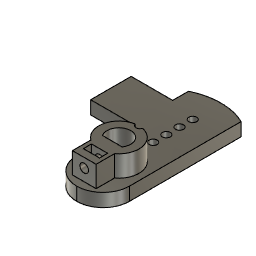
partA_5-1_geared v8 (Autodesk Fusion 360 design; units mm, degrees)
Autodesk Fusion 360 part; units mm, degrees
note: some values were not read from the file. Chosen so that the rebuilt part matches the saved one: which face or edge a step refers to. Set by a fixed rule: which sketch regions a step uses.
sketch "Sketch1" plane through (0, 0, 0) normal (0, 0, 1) x (1, 0, 0)
  circle A0 centre (19.9632, 20.0536) radius 32
  circle A1 centre (19.9632, 20.0536) radius 2.5692
  line L0 (16.8979, 9.6411) -> (23.0286, 9.6411)
  line L1 (23.0286, 9.6411) -> (23.0286, 12.7065)
  line L2 (23.0286, 12.7065) -> (16.8979, 12.7065)
  line L3 (16.8979, 12.7065) -> (16.8979, 9.6411)
  line L4 (18.9305, 17.7012) -> (20.996, 17.7012)
  circle A2 centre (20.0539, 47.9478) radius 1.5
  line L5 (19.9632, 20.0536) -> (20.0539, 47.9478) construction
  circle A3 centre (20.0539, 42.9478) radius 1.5
  circle A4 centre (20.0539, 37.9478) radius 1.5
  circle A5 centre (20.0539, 32.9478) radius 1.5
  circle A6 centre (20.0539, 27.9478) radius 1.5
  circle A7 centre (19.9632, 20.0536) radius 4.5
  line L6 (19.9779, 24.5536) -> (19.9551, 17.5536) construction
  line L7 (19.9551, 17.5536) -> (16.2135, 17.5658)
  line L8 (19.9551, 17.5536) -> (23.6968, 17.5415)
  dimension "d1" = 64
  dimension "d2" = 3
  dimension "d18" = 3
  dimension "d19" = 3
  dimension "d20" = 3
  dimension "d21" = 3
  dimension "d26" = 9
  dimension "d27" = 7
  constraint concentric A0 A1
  constraint horizontal L0
  constraint vertical L1
  constraint horizontal L2
  constraint vertical L3
  constraint coincident A1 L4.start
  constraint coincident A1 L4.end
  constraint horizontal L4
  constraint coincident A0.centre A1.centre
  constraint coincident A2.centre L5.end
  constraint concentric A0 A7
  constraint coincident A7 L6.start
  constraint coincident L5 L6.start
  constraint parallel L5 L6
  constraint coincident A7 L7.end
  constraint perpendicular L6 L7
  constraint coincident A7 L8.end
  constraint perpendicular L6 L8
  measures "d1" diameter of A0
  measures "d2" diameter of A2
  measures "d18" diameter of A3
  measures "d19" diameter of A4
  measures "d20" diameter of A5
  measures "d21" diameter of A6
  measures "d26" diameter of A7
  measures "d27" distance of L6.start L6.end
extrude "Extrude1" add sketch "Sketch1" along normal blind 5 contours A0 | A1 A7 L7 L8 | A1 L4 L7 L8 | A1 L7 L8 | A1 A7 L7 L8 | A3 | A4 | A5 | A6
sketch "Sketch2" plane through (0, 0, 5) normal (0, 0, 1) x (-1, 0, 0)
  line L0 (-20.996, -17.7012) -> (-18.9305, -17.7012)
  arc A0 (-20.996, -17.7012) -> (-18.9305, -17.7012) centre (-19.9632, -20.0536) ccw
  circle A1 centre (-20.0539, -47.9478) radius 1.5
  line L1 (-16.8979, -9.6411) -> (-16.8979, -12.7065)
  line L2 (-16.8979, -12.7065) -> (-23.0286, -12.7065)
  line L3 (-23.0286, -12.7065) -> (-23.0286, -9.6411)
  line L4 (-23.0286, -9.6411) -> (-16.8979, -9.6411)
  circle A2 centre (-19.9632, -20.0536) radius 32
  circle A3 centre (-19.9632, -20.0536) radius 7.6208
  line L5 (-15.4848, -13.8875) -> (-24.4668, -13.8875)
  line L6 (-24.4668, -13.8875) -> (-24.4668, -6.9024)
  line L7 (-24.4668, -6.9024) -> (-15.4848, -6.9024)
  line L8 (-15.4848, -6.9024) -> (-15.4848, -13.8875)
  line L9 (-16.8979, -12.7065) -> (-23.0286, -12.7065)
  line L10 (-23.0286, -12.7065) -> (-23.0286, -13.8875)
  line L11 (-23.0286, -13.8875) -> (-16.8979, -13.8875)
  line L12 (-16.8979, -13.8875) -> (-16.8979, -12.7065)
  constraint concentric A0 A3
  constraint horizontal L5
  constraint vertical L6
  constraint horizontal L7
  constraint vertical L8
  constraint coincident A3 L5.start
  constraint horizontal L9
  constraint vertical L10
  constraint horizontal L11
  constraint vertical L12
  constraint coincident L5 L10.end
  constraint coincident L3 L10.end
  constraint coincident L1.end L2.start
extrude "Extrude2" add sketch "Sketch2" along normal blind 10 contours L1 L3 L4 A3 L5 L6 L7 L8 L10 L12 | L1 L2 L3 L4 A3 L9 | L2 A3 L9 L12 | L2 A3 L5 L9 L10 L11 L12 | A3 L5 L12 | L2 A3 L9 L10 | A3 L5 L11 | A3 L5 L10
sketch "Sketch3" plane through (0, 6.9024, 0) normal (0, -1, 0) x (1, 0, 0)
  line L0 (15.4848, 5) -> (24.4668, 5)
  line L1 (24.4668, 5) -> (24.4668, 15)
  line L2 (24.4668, 15) -> (15.4848, 15)
  line L3 (15.4848, 15) -> (15.4848, 5)
  circle A0 centre (19.9584, 9.4906) radius 1.65
  dimension "d7" = 3.3
  measures "d7" diameter of A0
extrude "Extrude3" cut sketch "Sketch3" against normal up to surface (10.7988 mm away) contours A0
sketch "Sketch4" plane through (0, 0, 0) normal (0, 0, -1) x (1, 0, 0)
  line L0 (18.9305, -17.7012) -> (20.996, -17.7012)
  arc A0 (18.9305, -17.7012) -> (20.996, -17.7012) centre (19.9632, -20.0536) ccw
  circle A1 centre (20.0539, -47.9478) radius 1.5
  line L1 (16.8979, -12.7065) -> (16.8979, -9.6411)
  line L2 (16.8979, -9.6411) -> (23.0286, -9.6411)
  line L3 (23.0286, -9.6411) -> (23.0286, -12.7065)
  line L4 (23.0286, -12.7065) -> (16.8979, -12.7065)
  circle A2 centre (19.9632, -20.0536) radius 32
  line L5 (19.9632, -20.0536) -> (19.9632, -4.0536) construction
  line L6 (19.9632, -4.0536) -> (29.9632, -4.0536)
  line L7 (29.9632, -4.0536) -> (29.9333, -50.4608)
  line L8 (9.9632, -4.0536) -> (9.9932, -50.4608)
  line L9 (19.9632, -4.0536) -> (9.9632, -4.0536)
  dimension "d10" = 16
  dimension "d11" = 10
  constraint coincident A0.centre A2.centre
  constraint perpendicular L2 L5
  constraint perpendicular L5 L6
  constraint coincident A2 L7.end
  constraint symmetric L6.start L5 L9.start
  constraint symmetric L5 L6.end L8.start
  constraint symmetric L5 L7.end L8.end
  measures "d10" distance of A0.centre L5.end
  measures "d11" distance of L5.end L6.end
extrude "Extrude4" cut sketch "Sketch4" against normal blind 17 contours A2 L6 L7 L8 L9 picked at (14.6424, 1.0929)
fillet "Fillet1" radius 10 2 edges at (9.9632, 4.0536, 2.5) (29.9632, 4.0536, 2.5)
fillet "Fillet2" radius 4 2 edges at (29.9333, 50.4608, 2.5) (9.9932, 50.4608, 2.5)
extrude "Extrude5" cut sketch "Sketch1" along normal up to surface (5 mm away) contours A3 | A4 | A5 | A6
extrude "Extrude6" cut sketch "Sketch1" along normal blind 16 contours A6
extrude "Extrude7" cut sketch "Sketch1" along normal up to surface (15 mm away) contours A1 L4 | A1 A7 L7 L8 | A1 L4 L7 L8 picked at (16.6304, 18.132)
sketch "Sketch5" plane through (0, 0, 15) normal (0, 0, 1) x (-1, 0, 0)
  line L0 (-23.6968, -17.5415) -> (-16.2135, -17.5658)
  arc A0 (-23.6968, -17.5415) -> (-16.2135, -17.5658) centre (-19.9632, -20.0536) ccw
  arc A1 (-18.6069, -27.5528) -> (-21.4915, -27.5196) centre (-20.0539, -27.9478) ccw
  arc A2 (-18.6069, -27.5528) -> (-15.4848, -13.8875) centre (-19.9632, -20.0536) ccw
  line L1 (-15.4848, -13.8875) -> (-15.4848, -6.9024)
  line L2 (-15.4848, -6.9024) -> (-24.4668, -6.9024)
  line L3 (-24.4668, -6.9024) -> (-24.4668, -13.8875)
  line L4 (-24.4668, -13.8875) -> (-24.4417, -13.8875)
  arc A3 (-24.4417, -13.8875) -> (-21.4915, -27.5196) centre (-19.9632, -20.0536) ccw
  arc A4 (-17.9394, -12.7065) -> (-21.9871, -12.7065) centre (-19.9632, -20.0536) ccw
  line L5 (-17.9394, -12.7065) -> (-21.9871, -12.7065)
  line L6 (-17.9394, -12.7065) -> (-21.9871, -12.7065)
  arc A5 (-17.9394, -12.7065) -> (-21.9871, -12.7065) centre (-19.9632, -20.0536) ccw
  constraint coincident A4.start L5.start
  constraint coincident A4.end L5.end
extrude "Extrude8" add sketch "Sketch5" against normal blind 15 contours A4 L5 L6 A5
sketch "Sketch6" plane through (0, 0, 0) normal (0, 0, -1) x (1, 0, 0)
  line L0 (16.2135, -17.5658) -> (23.6968, -17.5415)
  arc A0 (16.2135, -17.5658) -> (23.6968, -17.5415) centre (19.9632, -20.0536) ccw
  circle A1 centre (20.0539, -37.9478) radius 1.5
  circle A2 centre (20.0539, -32.9478) radius 1.5
  circle A3 centre (20.0539, -42.9478) radius 1.5
  circle A4 centre (20.0539, -27.9478) radius 1.5
  arc A5 (9.9912, -47.4119) -> (13.138, -51.3173) centre (13.9912, -47.4093) ccw
  arc A6 (13.138, -51.3173) -> (26.7885, -51.3173) centre (19.9632, -20.0536) ccw
  arc A7 (26.7885, -51.3173) -> (29.9353, -47.4119) centre (25.9353, -47.4093) ccw
  line L1 (29.9353, -47.4119) -> (29.9568, -14.0601)
  arc A8 (29.9568, -14.0601) -> (19.9697, -4.0536) centre (19.9568, -14.0536) ccw
  arc A9 (19.9697, -4.0536) -> (9.9697, -14.0601) centre (19.9697, -14.0536) ccw
  line L2 (9.9697, -14.0601) -> (9.9912, -47.4119)
  line L3 (16.8979, -12.7065) -> (16.8979, -9.6411)
  line L4 (16.8979, -9.6411) -> (23.0286, -9.6411)
  line L5 (23.0286, -9.6411) -> (23.0286, -12.7065)
  line L6 (23.0286, -12.7065) -> (21.9871, -12.7065)
  arc A10 (21.9871, -12.7065) -> (17.9394, -12.7065) centre (19.9632, -20.0536) ccw
  line L7 (17.9394, -12.7065) -> (16.8979, -12.7065)
  circle A11 centre (20.0539, -47.9478) radius 1.5
  line L8 (16.8979, -9.6411) -> (23.0286, -9.6411)
  line L9 (23.0286, -9.6411) -> (23.0286, -12.7065)
  line L10 (23.0286, -12.7065) -> (16.8979, -12.7065)
  line L11 (16.8979, -12.7065) -> (16.8979, -9.6411)
  constraint horizontal L8
  constraint vertical L9
  constraint horizontal L10
  constraint vertical L11
  constraint coincident L5.end L6.start
  constraint coincident L3.end L4.start
extrude "Extrude9" cut sketch "Sketch6" against normal blind 17 contours L3 L4 L5 L6 A10 L7 L8 L9 L10 L11 | A10 L10
move_face "OffsetFaces1" offset -2 1 faces at (18.9361, 15.9379, 15)
sketch "Sketch7" plane through (29.9658, 0.0193, 0) normal (1, 0.000645, 0) x (-0.000645, 1, 0)
  line L0 (47.3926, 0) -> (47.3926, 5)
  line L1 (47.3926, 5) -> (14.0408, 5)
  line L2 (14.0408, 5) -> (14.0408, 0)
  line L3 (14.0408, 0) -> (47.3926, 0)
  line L4 (46.3289, 5) -> (35.3289, 5)
  line L5 (35.3289, 5) -> (35.3289, -0.8317)
  line L6 (35.3289, -0.8317) -> (46.3289, -0.8317)
  line L7 (46.3289, -0.8317) -> (46.3289, 5)
  dimension "d35" = 11
  constraint horizontal L4
  constraint vertical L5
  constraint horizontal L6
  constraint vertical L7
  constraint coincident L1 L4.start
  measures "d35" distance of L4.start L4.end
sketch "Sketch8" plane through (9.9606, -0.0064, 0) normal (-1, 0.000645, 0) x (-0.000645, -1, 0)
  line L0 (-47.4183, 5) -> (-47.4183, 0)
  line L1 (-47.4183, 0) -> (-14.0665, 0)
  line L2 (-14.0665, 0) -> (-14.0665, 5)
  line L3 (-14.0665, 5) -> (-47.4183, 5)
  line L4 (-53.3675, 5) -> (-35.0609, 5)
  line L5 (-35.0609, 5) -> (-35.0609, -1.1511)
  line L6 (-35.0609, -1.1511) -> (-53.3675, -1.1511)
  line L7 (-53.3675, -1.1511) -> (-53.3675, 5)
  point P0 (-47.4312, 5)
  point P1 (-14.0794, 5)
  constraint horizontal L4
  constraint vertical L5
  constraint horizontal L6
  constraint vertical L7
extrude "Extrude11" add sketch "Sketch8" along normal blind 15.75 contours L0 L1 L3 L4 L5
sketch "Sketch11" plane through (0, 0, 0) normal (0, 0, -1) x (1, 0, 0)
  line L0 (23.0286, -12.7065) -> (16.8979, -12.7065)
  line L1 (16.8979, -12.7065) -> (16.8979, -9.6411)
  line L2 (16.8979, -9.6411) -> (23.0286, -9.6411)
  line L3 (23.0286, -9.6411) -> (23.0286, -12.7065)
  line L4 (16.2135, -17.5658) -> (23.6968, -17.5415)
  arc A0 (16.2135, -17.5658) -> (23.6968, -17.5415) centre (19.9632, -20.0536) ccw
  circle A1 centre (20.0539, -37.9478) radius 1.5
  circle A2 centre (20.0539, -32.9478) radius 1.5
  circle A3 centre (20.0539, -42.9478) radius 1.5
  circle A4 centre (20.0539, -27.9478) radius 1.5
  arc A5 (9.9912, -47.4119) -> (13.138, -51.3173) centre (13.9912, -47.4093) ccw
  arc A6 (13.138, -51.3173) -> (26.7885, -51.3173) centre (19.9632, -20.0536) ccw
  arc A7 (26.7885, -51.3173) -> (29.9353, -47.4119) centre (25.9353, -47.4093) ccw
  line L5 (29.9353, -47.4119) -> (29.9568, -14.0601)
  arc A8 (29.9568, -14.0601) -> (19.9697, -4.0536) centre (19.9568, -14.0536) ccw
  arc A9 (19.9697, -4.0536) -> (9.9697, -14.0601) centre (19.9697, -14.0536) ccw
  line L6 (9.9697, -14.0601) -> (9.9832, -35.0545)
  line L7 (9.9832, -35.0545) -> (-5.7668, -35.0646)
  line L8 (-5.7668, -35.0646) -> (-5.7588, -47.4221)
  circle A10 centre (20.0539, -47.9478) radius 1.5
  line L9 (29.9353, -47.4119) -> (29.9295, -56.4119)
  line L10 (29.9353, -47.4119) -> (9.9912, -47.4119) construction
  line L11 (9.9912, -47.4119) -> (9.9912, -56.4119)
  arc A11 (9.9912, -56.4119) -> (29.9295, -56.4119) centre (19.9603, -35.7562) ccw
  line L12 (-5.7588, -47.4221) -> (9.9912, -47.4119)
  dimension "d46" = 9
  dimension "d48" = 9
  constraint coincident A7.end L5.start
  constraint parallel L5 L9
  constraint coincident A5.start L10.end
  constraint perpendicular L10 L11
  measures "d46" distance of A7.end L9.end
  measures "d48" distance of A5.start L11.end
extrude "Extrude14" add sketch "Sketch11" against normal blind 5 contours A5 A6 A7 L9 L11 A11
move_face "OffsetFaces3" offset 3 1 faces at (-0.5088, 47.4187, 1.6667)
